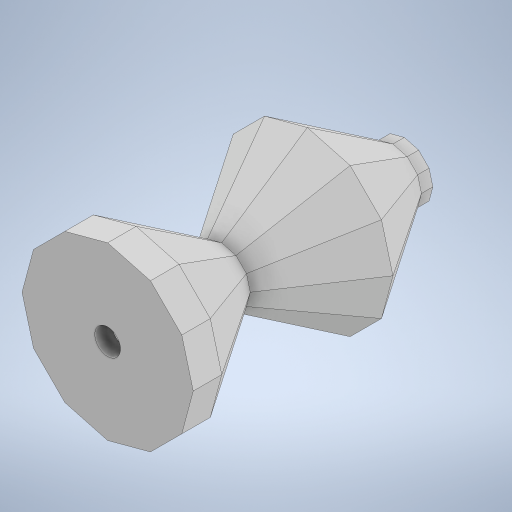
# Autodesk Inventor part: Test30.30
Saved by Autodesk Inventor 2023 (Build 270158000, 158)
## iProperties
Created: 2024-07-08
Part Number: Test30.30
Material: 일반
Document SubType Name: Modeling
Designer: ojs08
Density: 1 g/cm^3
Appearance: 기본값
Author: ojs08
Autodesk Inventor part; units mm, degrees
ref_plane "YZ Plane" through (0, 0, 0) normal (1, 0, 0) x (0, 1, 0)
ref_plane "XZ Plane" through (0, 0, 0) normal (0, 1, 0) x (-1, 0, 0)
sketch "스케치1" plane through (0, 0, 0) normal (0, 0, 1) x (1, 0, 0)
  line L0 (12.9904, -7.5) -> (7.5, -12.9904)
  line L1 (7.5, -12.9904) -> (0, -15)
  line L2 (0, -15) -> (-7.5, -12.9904)
  line L3 (-7.5, -12.9904) -> (-12.9904, -7.5)
  line L4 (-12.9904, -7.5) -> (-15, 0)
  line L5 (-15, 0) -> (-12.9904, 7.5)
  line L6 (-12.9904, 7.5) -> (-7.5, 12.9904)
  line L7 (-7.5, 12.9904) -> (0, 15)
  line L8 (0, 15) -> (7.5, 12.9904)
  line L9 (7.5, 12.9904) -> (12.9904, 7.5)
  line L10 (12.9904, 7.5) -> (15, 0)
  line L11 (15, 0) -> (12.9904, -7.5)
  line L12 (-21, 0) -> (21, 0) projected
  point P0 (0, 0)
  point P1 (0, 0)
  dimension "d0" = 30
  constraints: 24 end point, 1 coincident, 1 point on line, 25 other
  measures "d0" distance of L10.end L4.end
ref_plane "작업 평면1" through (0, 0, 15) normal (0, 0, 1) x (1, 0, 0)
sketch "스케치2" plane through (0, 0, 15) normal (0, 0, 1) x (1, 0, 0)
  line L0 (2.5, -4.3301) -> (0, -5)
  line L1 (0, -5) -> (-2.5, -4.3301)
  line L2 (-2.5, -4.3301) -> (-4.3301, -2.5)
  line L3 (-4.3301, -2.5) -> (-5, 0)
  line L4 (-5, 0) -> (-4.3301, 2.5)
  line L5 (-4.3301, 2.5) -> (-2.5, 4.3301)
  line L6 (-2.5, 4.3301) -> (0, 5)
  line L7 (0, 5) -> (2.5, 4.3301)
  line L8 (2.5, 4.3301) -> (4.3301, 2.5)
  line L9 (4.3301, 2.5) -> (5, 0)
  line L10 (5, 0) -> (4.3301, -2.5)
  line L11 (4.3301, -2.5) -> (2.5, -4.3301)
  line L12 (-21, 0) -> (21, 0) projected
  point P0 (0, 0)
  point P1 (0, 0)
  dimension "d2" = 10
  constraints: 24 end point, 1 coincident, 1 point on line, 25 other
  measures "d2" distance of L9.end L3.end
loft "로프트1" add profiles "스케치1", "스케치2"
mirror "미러1" about plane through (0, 0, 15) normal (0, 0, 1) of "로프트1"
mirror "미러2" about plane through (0, 0, 0) normal (0, 0, -1) of "로프트1"
sketch "스케치3" plane through (7.5, -12.9904, 30) normal (0, 0, 1) x (0.7071068, -0.7071068, 0)
  line L0 (0, 7.7646) -> (0, 0) projected
  line L1 (-3.8823, 14.4889) -> (0, 7.7646) projected
  line L2 (-10.6066, 18.3712) -> (-3.8823, 14.4889) projected
  line L3 (-18.3712, 18.3712) -> (-10.6066, 18.3712) projected
  line L4 (-25.0955, 14.4889) -> (-18.3712, 18.3712) projected
  line L5 (-28.9778, 7.7646) -> (-25.0955, 14.4889) projected
  line L6 (-28.9778, 0) -> (-28.9778, 7.7646) projected
  line L7 (-25.0955, -6.7243) -> (-28.9778, 0) projected
  line L8 (-18.3712, -10.6066) -> (-25.0955, -6.7243) projected
  line L9 (-10.6066, -10.6066) -> (-18.3712, -10.6066) projected
  line L10 (-3.8823, -6.7243) -> (-10.6066, -10.6066) projected
  line L11 (0, 0) -> (-3.8823, -6.7243) projected
  point P0 (-14.4889, 3.8823)
extrude "돌출1" add sketch "스케치3" along normal blind 2.5
shell "쉘1" thickness 0.5 removed faces 0 ; own thickness 2 on faces at (3.3333, 12.4402, -2.5) (9.1068, 9.1068, -2.5) (12.4402, -3.3333, -2.5) (12.4402, 3.3333, -2.5) (9.1068, -9.1068, -2.5) (3.3333, -12.4402, -2.5) (-3.3333, -12.4402, -2.5) (-3.3333, 12.4402, -2.5) (-9.1068, 9.1068, -2.5) (-12.4402, 3.3333, -2.5) (-12.4402, -3.3333, -2.5) (-9.1068, -9.1068, -2.5) (9.1068, -9.1068, 27.5) (3.3333, -12.4402, 27.5) (12.4402, -3.3333, 27.5) (12.4402, 3.3333, 27.5) (9.1068, 9.1068, 27.5) (3.3333, 12.4402, 27.5) (-3.3333, 12.4402, 27.5) (-9.1068, 9.1068, 27.5) (-12.4402, 3.3333, 27.5) (-12.4402, -3.3333, 27.5) (-9.1068, -9.1068, 27.5) (-3.3333, -12.4402, 27.5)
sketch "스케치4" plane through (7.5, -12.9904, 32.5) normal (0, 0, 1) x (0.7071068, 0.7071068, 0)
  line L0 (14.4889, 3.8823) -> (18.3712, 10.6066) projected
  line L1 (18.3712, 10.6066) -> (18.3712, 18.3712) projected
  line L2 (18.3712, 18.3712) -> (14.4889, 25.0955) projected
  line L3 (14.4889, 25.0955) -> (7.7646, 28.9778) projected
  line L4 (7.7646, 28.9778) -> (0, 28.9778) projected
  line L5 (0, 28.9778) -> (-6.7243, 25.0955) projected
  line L6 (-6.7243, 25.0955) -> (-10.6066, 18.3712) projected
  line L7 (-10.6066, 18.3712) -> (-10.6066, 10.6066) projected
  line L8 (-10.6066, 10.6066) -> (-6.7243, 3.8823) projected
  line L9 (-6.7243, 3.8823) -> (0, 0) projected
  line L10 (0, 0) -> (7.7646, 0) projected
  line L11 (7.7646, 0) -> (14.4889, 3.8823) projected
  point P0 (3.8823, 14.4889)
extrude "돌출2" add sketch "스케치4" along normal blind 2.5
sketch "스케치5" plane through (7.5, -12.9904, 35) normal (0, 0, 1) x (0.7071068, -0.7071068, 0)
  circle A0 centre (-14.4889, 3.8823) radius 2.25
  dimension "d13" = 4.5
  constraints: 1 centre point, 1 coincident
  measures "d13" diameter of A0
extrude "돌출3" cut sketch "스케치5" against normal blind 3
sketch "스케치6" plane through (2.5, -4.3301, -15) normal (0, 0, -1) x (-0.7071068, 0.7071068, 0)
  line L0 (0, 2.5882) -> (0, 0) projected
  line L1 (0, 0) -> (1.2941, -2.2414) projected
  line L2 (1.2941, -2.2414) -> (3.5355, -3.5355) projected
  line L3 (3.5355, -3.5355) -> (6.1237, -3.5355) projected
  line L4 (6.1237, -3.5355) -> (8.3652, -2.2414) projected
  line L5 (8.3652, -2.2414) -> (9.6593, 0) projected
  line L6 (9.6593, 0) -> (9.6593, 2.5882) projected
  line L7 (9.6593, 2.5882) -> (8.3652, 4.8296) projected
  line L8 (8.3652, 4.8296) -> (6.1237, 6.1237) projected
  line L9 (6.1237, 6.1237) -> (3.5355, 6.1237) projected
  line L10 (3.5355, 6.1237) -> (1.2941, 4.8296) projected
  line L11 (1.2941, 4.8296) -> (0, 2.5882) projected
  point P0 (4.8296, 1.2941)
extrude "돌출4" add sketch "스케치6" along normal blind 2
